Autodesk Fusion 360 part; units mm, degrees
(part 8 of 40)
  line L3316 (187.8528, 216.8887) -> (187.8788, 217.0208) construction
  line L3317 (187.8788, 217.0208) -> (187.8986, 217.1199) construction
  line L3318 (187.8986, 217.1199) -> (187.912, 217.186) construction
  line L3319 (187.912, 217.186) -> (187.9188, 217.2191) construction
  arc A105 (192.2105, 218.6136) -> (187.9188, 217.2191) centre (212.132, 150) ccw
  arc A106 (192.2105, 218.6136) -> (187.9188, 217.2191) centre (212.132, 150) ccw
  line L3320 (271.2762, 155.5428) -> (272.9005, 155.6951)
  spline S44 degree 5 poles (206.4369, 89.2315) (206.4341, 89.2007) (206.4291, 89.1391) (206.4242, 89.0467) (206.4223, 88.9234) (206.4264, 88.769) (206.4351, 88.6144) (206.4466, 88.4597) (206.4597, 88.305) (206.4737, 88.1502) (206.4889, 87.9955) (206.5055, 87.8407) (206.524, 87.686) (206.5449, 87.5312) (206.5679, 87.3765) (206.593, 87.2218) (206.6199, 87.0671) (206.6482, 86.9125) (206.6778, 86.7579) (206.7087, 86.6034) (206.7407, 86.4489) (206.7741, 86.2945) (206.8088, 86.1402) (206.8449, 85.986) (206.8823, 85.8318) (206.9211, 85.6778) (206.9611, 85.5238) (207.0023, 85.3699) (207.0447, 85.2161) (207.0881, 85.0624) (207.1327, 84.9088) (207.1784, 84.7553) (207.2252, 84.602) (207.2731, 84.4487) (207.3221, 84.2956) (207.3721, 84.1426) (207.4233, 83.9897) (207.4754, 83.8369) (207.5285, 83.6842) (207.5827, 83.5317) (207.6378, 83.3794) (207.694, 83.2271) (207.751, 83.075) (207.8091, 82.923) (207.8681, 82.7712) (207.9281, 82.6196) (207.989, 82.468) (208.0508, 82.3167) (208.1135, 82.1655) (208.1772, 82.0144) (208.2417, 81.8635) (208.3071, 81.7128) (208.3735, 81.5622) (208.4407, 81.4118) (208.5087, 81.2616) (208.5777, 81.1115) (208.6474, 80.9616) (208.7181, 80.8119) (208.7895, 80.6624) (208.8619, 80.513) (208.935, 80.3638) (209.009, 80.2148) (209.0838, 80.066) (209.1594, 79.9174) (209.2358, 79.7689) (209.313, 79.6207) (209.391, 79.4726) (209.4698, 79.3248) (209.5494, 79.1771) (209.6297, 79.0297) (209.7109, 78.8824) (209.7764, 78.7648) (209.8259, 78.6766) (209.8591, 78.6179) (209.8757, 78.5885) knots 0 0 0 0 0 0 0.01428571 0.02857143 0.04285714 0.05714286 0.07142857 0.08571429 0.1 0.11428571 0.12857143 0.14285714 0.15714286 0.17142857 0.18571429 0.2 0.21428571 0.22857143 0.24285714 0.25714286 0.27142857 0.28571429 0.3 0.31428571 0.32857143 0.34285714 0.35714286 0.37142857 0.38571429 0.4 0.41428571 0.42857143 0.44285714 0.45714286 0.47142857 0.48571429 0.5 0.51428571 0.52857143 0.54285714 0.55714286 0.57142857 0.58571429 0.6 0.61428571 0.62857143 0.64285714 0.65714286 0.67142857 0.68571429 0.7 0.71428571 0.72857143 0.74285714 0.75714286 0.77142857 0.78571429 0.8 0.81428571 0.82857143 0.84285714 0.85714286 0.87142857 0.88571429 0.9 0.91428571 0.92857143 0.94285714 0.95714286 0.97142857 0.98571429 1 1 1 1 1 1
  line L3321 (206.4369, 89.2315) -> (206.4341, 89.2007) construction
  line L3322 (206.4341, 89.2007) -> (206.4291, 89.1391) construction
  line L3323 (206.4291, 89.1391) -> (206.4242, 89.0467) construction
  line L3324 (206.4242, 89.0467) -> (206.4223, 88.9234) construction
  line L3325 (206.4223, 88.9234) -> (206.4264, 88.769) construction
  line L3326 (206.4264, 88.769) -> (206.4351, 88.6144) construction
  line L3327 (206.4351, 88.6144) -> (206.4466, 88.4597) construction
  line L3328 (206.4466, 88.4597) -> (206.4597, 88.305) construction
  line L3329 (206.4597, 88.305) -> (206.4737, 88.1502) construction
  line L3330 (206.4737, 88.1502) -> (206.4889, 87.9955) construction
  line L3331 (206.4889, 87.9955) -> (206.5055, 87.8407) construction
  line L3332 (206.5055, 87.8407) -> (206.524, 87.686) construction
  line L3333 (206.524, 87.686) -> (206.5449, 87.5312) construction
  line L3334 (206.5449, 87.5312) -> (206.5679, 87.3765) construction
  line L3335 (206.5679, 87.3765) -> (206.593, 87.2218) construction
  line L3336 (206.593, 87.2218) -> (206.6199, 87.0671) construction
  line L3337 (206.6199, 87.0671) -> (206.6482, 86.9125) construction
  line L3338 (206.6482, 86.9125) -> (206.6778, 86.7579) construction
  line L3339 (206.6778, 86.7579) -> (206.7087, 86.6034) construction
  line L3340 (206.7087, 86.6034) -> (206.7407, 86.4489) construction
  line L3341 (206.7407, 86.4489) -> (206.7741, 86.2945) construction
  line L3342 (206.7741, 86.2945) -> (206.8088, 86.1402) construction
  line L3343 (206.8088, 86.1402) -> (206.8449, 85.986) construction
  line L3344 (206.8449, 85.986) -> (206.8823, 85.8318) construction
  line L3345 (206.8823, 85.8318) -> (206.9211, 85.6778) construction
  line L3346 (206.9211, 85.6778) -> (206.9611, 85.5238) construction
  line L3347 (206.9611, 85.5238) -> (207.0023, 85.3699) construction
  line L3348 (207.0023, 85.3699) -> (207.0447, 85.2161) construction
  line L3349 (207.0447, 85.2161) -> (207.0881, 85.0624) construction
  line L3350 (207.0881, 85.0624) -> (207.1327, 84.9088) construction
  line L3351 (207.1327, 84.9088) -> (207.1784, 84.7553) construction
  line L3352 (207.1784, 84.7553) -> (207.2252, 84.602) construction
  line L3353 (207.2252, 84.602) -> (207.2731, 84.4487) construction
  line L3354 (207.2731, 84.4487) -> (207.3221, 84.2956) construction
  line L3355 (207.3221, 84.2956) -> (207.3721, 84.1426) construction
  line L3356 (207.3721, 84.1426) -> (207.4233, 83.9897) construction
  line L3357 (207.4233, 83.9897) -> (207.4754, 83.8369) construction
  line L3358 (207.4754, 83.8369) -> (207.5285, 83.6842) construction
  line L3359 (207.5285, 83.6842) -> (207.5827, 83.5317) construction
  line L3360 (207.5827, 83.5317) -> (207.6378, 83.3794) construction
  line L3361 (207.6378, 83.3794) -> (207.694, 83.2271) construction
  line L3362 (207.694, 83.2271) -> (207.751, 83.075) construction
  line L3363 (207.751, 83.075) -> (207.8091, 82.923) construction
  line L3364 (207.8091, 82.923) -> (207.8681, 82.7712) construction
  line L3365 (207.8681, 82.7712) -> (207.9281, 82.6196) construction
  line L3366 (207.9281, 82.6196) -> (207.989, 82.468) construction
  line L3367 (207.989, 82.468) -> (208.0508, 82.3167) construction
  line L3368 (208.0508, 82.3167) -> (208.1135, 82.1655) construction
  line L3369 (208.1135, 82.1655) -> (208.1772, 82.0144) construction
  line L3370 (208.1772, 82.0144) -> (208.2417, 81.8635) construction
  line L3371 (208.2417, 81.8635) -> (208.3071, 81.7128) construction
  line L3372 (208.3071, 81.7128) -> (208.3735, 81.5622) construction
  line L3373 (208.3735, 81.5622) -> (208.4407, 81.4118) construction
  line L3374 (208.4407, 81.4118) -> (208.5087, 81.2616) construction
  line L3375 (208.5087, 81.2616) -> (208.5777, 81.1115) construction
  line L3376 (208.5777, 81.1115) -> (208.6474, 80.9616) construction
  line L3377 (208.6474, 80.9616) -> (208.7181, 80.8119) construction
  line L3378 (208.7181, 80.8119) -> (208.7895, 80.6624) construction
  line L3379 (208.7895, 80.6624) -> (208.8619, 80.513) construction
  line L3380 (208.8619, 80.513) -> (208.935, 80.3638) construction
  line L3381 (208.935, 80.3638) -> (209.009, 80.2148) construction
  line L3382 (209.009, 80.2148) -> (209.0838, 80.066) construction
  line L3383 (209.0838, 80.066) -> (209.1594, 79.9174) construction
  line L3384 (209.1594, 79.9174) -> (209.2358, 79.7689) construction
  line L3385 (209.2358, 79.7689) -> (209.313, 79.6207) construction
  line L3386 (209.313, 79.6207) -> (209.391, 79.4726) construction
  line L3387 (209.391, 79.4726) -> (209.4698, 79.3248) construction
  line L3388 (209.4698, 79.3248) -> (209.5494, 79.1771) construction
  line L3389 (209.5494, 79.1771) -> (209.6297, 79.0297) construction
  line L3390 (209.6297, 79.0297) -> (209.7109, 78.8824) construction
  line L3391 (209.7109, 78.8824) -> (209.7764, 78.7648) construction
  line L3392 (209.7764, 78.7648) -> (209.8259, 78.6766) construction
  line L3393 (209.8259, 78.6766) -> (209.8591, 78.6179) construction
  line L3394 (209.8591, 78.6179) -> (209.8757, 78.5885) construction
  spline S45 degree 5 poles (206.4369, 89.2315) (206.4341, 89.2007) (206.4291, 89.1391) (206.4242, 89.0467) (206.4223, 88.9234) (206.4264, 88.769) (206.4351, 88.6144) (206.4466, 88.4597) (206.4597, 88.305) (206.4737, 88.1502) (206.4889, 87.9955) (206.5055, 87.8407) (206.524, 87.686) (206.5449, 87.5312) (206.5679, 87.3765) (206.593, 87.2218) (206.6199, 87.0671) (206.6482, 86.9125) (206.6778, 86.7579) (206.7087, 86.6034) (206.7407, 86.4489) (206.7741, 86.2945) (206.8088, 86.1402) (206.8449, 85.986) (206.8823, 85.8318) (206.9211, 85.6778) (206.9611, 85.5238) (207.0023, 85.3699) (207.0447, 85.2161) (207.0881, 85.0624) (207.1327, 84.9088) (207.1784, 84.7553) (207.2252, 84.602) (207.2731, 84.4487) (207.3221, 84.2956) (207.3721, 84.1426) (207.4233, 83.9897) (207.4754, 83.8369) (207.5285, 83.6842) (207.5827, 83.5317) (207.6378, 83.3794) (207.694, 83.2271) (207.751, 83.075) (207.8091, 82.923) (207.8681, 82.7712) (207.9281, 82.6196) (207.989, 82.468) (208.0508, 82.3167) (208.1135, 82.1655) (208.1772, 82.0144) (208.2417, 81.8635) (208.3071, 81.7128) (208.3735, 81.5622) (208.4407, 81.4118) (208.5087, 81.2616) (208.5777, 81.1115) (208.6474, 80.9616) (208.7181, 80.8119) (208.7895, 80.6624) (208.8619, 80.513) (208.935, 80.3638) (209.009, 80.2148) (209.0838, 80.066) (209.1594, 79.9174) (209.2358, 79.7689) (209.313, 79.6207) (209.391, 79.4726) (209.4698, 79.3248) (209.5494, 79.1771) (209.6297, 79.0297) (209.7109, 78.8824) (209.7764, 78.7648) (209.8259, 78.6766) (209.8591, 78.6179) (209.8757, 78.5885) knots 0 0 0 0 0 0 0.01428571 0.02857143 0.04285714 0.05714286 0.07142857 0.08571429 0.1 0.11428571 0.12857143 0.14285714 0.15714286 0.17142857 0.18571429 0.2 0.21428571 0.22857143 0.24285714 0.25714286 0.27142857 0.28571429 0.3 0.31428571 0.32857143 0.34285714 0.35714286 0.37142857 0.38571429 0.4 0.41428571 0.42857143 0.44285714 0.45714286 0.47142857 0.48571429 0.5 0.51428571 0.52857143 0.54285714 0.55714286 0.57142857 0.58571429 0.6 0.61428571 0.62857143 0.64285714 0.65714286 0.67142857 0.68571429 0.7 0.71428571 0.72857143 0.74285714 0.75714286 0.77142857 0.78571429 0.8 0.81428571 0.82857143 0.84285714 0.85714286 0.87142857 0.88571429 0.9 0.91428571 0.92857143 0.94285714 0.95714286 0.97142857 0.98571429 1 1 1 1 1 1
  line L3395 (206.4369, 89.2315) -> (206.4341, 89.2007) construction
  line L3396 (206.4341, 89.2007) -> (206.4291, 89.1391) construction
  line L3397 (206.4291, 89.1391) -> (206.4242, 89.0467) construction
  line L3398 (206.4242, 89.0467) -> (206.4223, 88.9234) construction
  line L3399 (206.4223, 88.9234) -> (206.4264, 88.769) construction
  line L3400 (206.4264, 88.769) -> (206.4351, 88.6144) construction
  line L3401 (206.4351, 88.6144) -> (206.4466, 88.4597) construction
  line L3402 (206.4466, 88.4597) -> (206.4597, 88.305) construction
  line L3403 (206.4597, 88.305) -> (206.4737, 88.1502) construction
  line L3404 (206.4737, 88.1502) -> (206.4889, 87.9955) construction
  line L3405 (206.4889, 87.9955) -> (206.5055, 87.8407) construction
  line L3406 (206.5055, 87.8407) -> (206.524, 87.686) construction
  line L3407 (206.524, 87.686) -> (206.5449, 87.5312) construction
  line L3408 (206.5449, 87.5312) -> (206.5679, 87.3765) construction
  line L3409 (206.5679, 87.3765) -> (206.593, 87.2218) construction
  line L3410 (206.593, 87.2218) -> (206.6199, 87.0671) construction
  line L3411 (206.6199, 87.0671) -> (206.6482, 86.9125) construction
  line L3412 (206.6482, 86.9125) -> (206.6778, 86.7579) construction
  line L3413 (206.6778, 86.7579) -> (206.7087, 86.6034) construction
  line L3414 (206.7087, 86.6034) -> (206.7407, 86.4489) construction
  line L3415 (206.7407, 86.4489) -> (206.7741, 86.2945) construction
  line L3416 (206.7741, 86.2945) -> (206.8088, 86.1402) construction
  line L3417 (206.8088, 86.1402) -> (206.8449, 85.986) construction
  line L3418 (206.8449, 85.986) -> (206.8823, 85.8318) construction
  line L3419 (206.8823, 85.8318) -> (206.9211, 85.6778) construction
  line L3420 (206.9211, 85.6778) -> (206.9611, 85.5238) construction
  line L3421 (206.9611, 85.5238) -> (207.0023, 85.3699) construction
  line L3422 (207.0023, 85.3699) -> (207.0447, 85.2161) construction
  line L3423 (207.0447, 85.2161) -> (207.0881, 85.0624) construction
  line L3424 (207.0881, 85.0624) -> (207.1327, 84.9088) construction
  line L3425 (207.1327, 84.9088) -> (207.1784, 84.7553) construction
  line L3426 (207.1784, 84.7553) -> (207.2252, 84.602) construction
  line L3427 (207.2252, 84.602) -> (207.2731, 84.4487) construction
  line L3428 (207.2731, 84.4487) -> (207.3221, 84.2956) construction
  line L3429 (207.3221, 84.2956) -> (207.3721, 84.1426) construction
  line L3430 (207.3721, 84.1426) -> (207.4233, 83.9897) construction
  line L3431 (207.4233, 83.9897) -> (207.4754, 83.8369) construction
  line L3432 (207.4754, 83.8369) -> (207.5285, 83.6842) construction
  line L3433 (207.5285, 83.6842) -> (207.5827, 83.5317) construction
  line L3434 (207.5827, 83.5317) -> (207.6378, 83.3794) construction
  line L3435 (207.6378, 83.3794) -> (207.694, 83.2271) construction
  line L3436 (207.694, 83.2271) -> (207.751, 83.075) construction
  line L3437 (207.751, 83.075) -> (207.8091, 82.923) construction
  line L3438 (207.8091, 82.923) -> (207.8681, 82.7712) construction
  line L3439 (207.8681, 82.7712) -> (207.9281, 82.6196) construction
  line L3440 (207.9281, 82.6196) -> (207.989, 82.468) construction
  line L3441 (207.989, 82.468) -> (208.0508, 82.3167) construction
  line L3442 (208.0508, 82.3167) -> (208.1135, 82.1655) construction
  line L3443 (208.1135, 82.1655) -> (208.1772, 82.0144) construction
  line L3444 (208.1772, 82.0144) -> (208.2417, 81.8635) construction
  line L3445 (208.2417, 81.8635) -> (208.3071, 81.7128) construction
  line L3446 (208.3071, 81.7128) -> (208.3735, 81.5622) construction
  line L3447 (208.3735, 81.5622) -> (208.4407, 81.4118) construction
  line L3448 (208.4407, 81.4118) -> (208.5087, 81.2616) construction
  line L3449 (208.5087, 81.2616) -> (208.5777, 81.1115) construction
  line L3450 (208.5777, 81.1115) -> (208.6474, 80.9616) construction
  line L3451 (208.6474, 80.9616) -> (208.7181, 80.8119) construction
  line L3452 (208.7181, 80.8119) -> (208.7895, 80.6624) construction
  line L3453 (208.7895, 80.6624) -> (208.8619, 80.513) construction
  line L3454 (208.8619, 80.513) -> (208.935, 80.3638) construction
  line L3455 (208.935, 80.3638) -> (209.009, 80.2148) construction
  line L3456 (209.009, 80.2148) -> (209.0838, 80.066) construction
  line L3457 (209.0838, 80.066) -> (209.1594, 79.9174) construction
  line L3458 (209.1594, 79.9174) -> (209.2358, 79.7689) construction
  line L3459 (209.2358, 79.7689) -> (209.313, 79.6207) construction
  line L3460 (209.313, 79.6207) -> (209.391, 79.4726) construction
  line L3461 (209.391, 79.4726) -> (209.4698, 79.3248) construction
  line L3462 (209.4698, 79.3248) -> (209.5494, 79.1771) construction
  line L3463 (209.5494, 79.1771) -> (209.6297, 79.0297) construction
  line L3464 (209.6297, 79.0297) -> (209.7109, 78.8824) construction
  line L3465 (209.7109, 78.8824) -> (209.7764, 78.7648) construction
  line L3466 (209.7764, 78.7648) -> (209.8259, 78.6766) construction
  line L3467 (209.8259, 78.6766) -> (209.8591, 78.6179) construction
  line L3468 (209.8591, 78.6179) -> (209.8757, 78.5885) construction
  arc A107 (209.8757, 78.5885) -> (214.3883, 78.5885) centre (212.132, 150) ccw
  arc A108 (209.8757, 78.5885) -> (214.3883, 78.5885) centre (212.132, 150) ccw
  spline S46 degree 5 poles (252.4583, 104.1847) (252.4787, 104.1615) (252.5188, 104.1146) (252.5771, 104.0427) (252.6512, 103.944) (252.7386, 103.8167) (252.8224, 103.6865) (252.904, 103.5546) (252.9844, 103.4218) (253.064, 103.2883) (253.1427, 103.1542) (253.2203, 103.0193) (253.2962, 102.8832) (253.3703, 102.7457) (253.4426, 102.607) (253.5133, 102.4671) (253.5824, 102.3262) (253.6504, 102.1844) (253.7173, 102.0419) (253.7832, 101.8988) (253.848, 101.755) (253.9118, 101.6105) (253.9744, 101.4653) (254.0359, 101.3193) (254.0962, 101.1726) (254.1554, 101.0251) (254.2135, 100.877) (254.2706, 100.7283) (254.3267, 100.579) (254.3819, 100.4291) (254.4361, 100.2786) (254.4894, 100.1276) (254.5417, 99.976) (254.593, 99.8239) (254.6434, 99.6712) (254.6928, 99.518) (254.7414, 99.3642) (254.789, 99.21) (254.8357, 99.0553) (254.8815, 98.9001) (254.9265, 98.7444) (254.9706, 98.5882) (255.0138, 98.4316) (255.0561, 98.2745) (255.0976, 98.117) (255.1383, 97.9591) (255.1781, 97.8007) (255.217, 97.6419) (255.2551, 97.4827) (255.2924, 97.3231) (255.3289, 97.1631) (255.3646, 97.0027) (255.3994, 96.8419) (255.4335, 96.6807) (255.4667, 96.5191) (255.4992, 96.3572) (255.5308, 96.1949) (255.5617, 96.0323) (255.5917, 95.8693) (255.621, 95.706) (255.6495, 95.5423) (255.6773, 95.3783) (255.7043, 95.2139) (255.7304, 95.0492) (255.7559, 94.8842) (255.7806, 94.7189) (255.8045, 94.5533) (255.8276, 94.3874) (255.85, 94.2211) (255.8717, 94.0546) (255.8926, 93.8878) (255.9087, 93.7541) (255.9205, 93.6537) (255.9282, 93.5867) (255.932, 93.5531) knots 0 0 0 0 0 0 0.01428571 0.02857143 0.04285714 0.05714286 0.07142857 0.08571429 0.1 0.11428571 0.12857143 0.14285714 0.15714286 0.17142857 0.18571429 0.2 0.21428571 0.22857143 0.24285714 0.25714286 0.27142857 0.28571429 0.3 0.31428571 0.32857143 0.34285714 0.35714286 0.37142857 0.38571429 0.4 0.41428571 0.42857143 0.44285714 0.45714286 0.47142857 0.48571429 0.5 0.51428571 0.52857143 0.54285714 0.55714286 0.57142857 0.58571429 0.6 0.61428571 0.62857143 0.64285714 0.65714286 0.67142857 0.68571429 0.7 0.71428571 0.72857143 0.74285714 0.75714286 0.77142857 0.78571429 0.8 0.81428571 0.82857143 0.84285714 0.85714286 0.87142857 0.88571429 0.9 0.91428571 0.92857143 0.94285714 0.95714286 0.97142857 0.98571429 1 1 1 1 1 1
  line L3469 (252.4583, 104.1847) -> (252.4787, 104.1615) construction
  line L3470 (252.4787, 104.1615) -> (252.5188, 104.1146) construction
  line L3471 (252.5188, 104.1146) -> (252.5771, 104.0427) construction
  line L3472 (252.5771, 104.0427) -> (252.6512, 103.944) construction
  line L3473 (252.6512, 103.944) -> (252.7386, 103.8167) construction
  line L3474 (252.7386, 103.8167) -> (252.8224, 103.6865) construction
  line L3475 (252.8224, 103.6865) -> (252.904, 103.5546) construction
  line L3476 (252.904, 103.5546) -> (252.9844, 103.4218) construction
  line L3477 (252.9844, 103.4218) -> (253.064, 103.2883) construction
  line L3478 (253.064, 103.2883) -> (253.1427, 103.1542) construction
  line L3479 (253.1427, 103.1542) -> (253.2203, 103.0193) construction
  line L3480 (253.2203, 103.0193) -> (253.2962, 102.8832) construction
  line L3481 (253.2962, 102.8832) -> (253.3703, 102.7457) construction
  line L3482 (253.3703, 102.7457) -> (253.4426, 102.607) construction
  line L3483 (253.4426, 102.607) -> (253.5133, 102.4671) construction
  line L3484 (253.5133, 102.4671) -> (253.5824, 102.3262) construction
  line L3485 (253.5824, 102.3262) -> (253.6504, 102.1844) construction
  line L3486 (253.6504, 102.1844) -> (253.7173, 102.0419) construction
  line L3487 (253.7173, 102.0419) -> (253.7832, 101.8988) construction
  line L3488 (253.7832, 101.8988) -> (253.848, 101.755) construction
  line L3489 (253.848, 101.755) -> (253.9118, 101.6105) construction
  line L3490 (253.9118, 101.6105) -> (253.9744, 101.4653) construction
  line L3491 (253.9744, 101.4653) -> (254.0359, 101.3193) construction
  line L3492 (254.0359, 101.3193) -> (254.0962, 101.1726) construction
  line L3493 (254.0962, 101.1726) -> (254.1554, 101.0251) construction
  line L3494 (254.1554, 101.0251) -> (254.2135, 100.877) construction
  line L3495 (254.2135, 100.877) -> (254.2706, 100.7283) construction
  line L3496 (254.2706, 100.7283) -> (254.3267, 100.579) construction
  line L3497 (254.3267, 100.579) -> (254.3819, 100.4291) construction
  line L3498 (254.3819, 100.4291) -> (254.4361, 100.2786) construction
  line L3499 (254.4361, 100.2786) -> (254.4894, 100.1276) construction
  line L3500 (254.4894, 100.1276) -> (254.5417, 99.976) construction
  line L3501 (254.5417, 99.976) -> (254.593, 99.8239) construction
  line L3502 (254.593, 99.8239) -> (254.6434, 99.6712) construction
  line L3503 (254.6434, 99.6712) -> (254.6928, 99.518) construction
  line L3504 (254.6928, 99.518) -> (254.7414, 99.3642) construction
  line L3505 (254.7414, 99.3642) -> (254.789, 99.21) construction
  line L3506 (254.789, 99.21) -> (254.8357, 99.0553) construction
  line L3507 (254.8357, 99.0553) -> (254.8815, 98.9001) construction
  line L3508 (254.8815, 98.9001) -> (254.9265, 98.7444) construction
  line L3509 (254.9265, 98.7444) -> (254.9706, 98.5882) construction
  line L3510 (254.9706, 98.5882) -> (255.0138, 98.4316) construction
  line L3511 (255.0138, 98.4316) -> (255.0561, 98.2745) construction
  line L3512 (255.0561, 98.2745) -> (255.0976, 98.117) construction
  line L3513 (255.0976, 98.117) -> (255.1383, 97.9591) construction
  line L3514 (255.1383, 97.9591) -> (255.1781, 97.8007) construction
  line L3515 (255.1781, 97.8007) -> (255.217, 97.6419) construction
  line L3516 (255.217, 97.6419) -> (255.2551, 97.4827) construction
  line L3517 (255.2551, 97.4827) -> (255.2924, 97.3231) construction
  line L3518 (255.2924, 97.3231) -> (255.3289, 97.1631) construction
  line L3519 (255.3289, 97.1631) -> (255.3646, 97.0027) construction
  line L3520 (255.3646, 97.0027) -> (255.3994, 96.8419) construction
  line L3521 (255.3994, 96.8419) -> (255.4335, 96.6807) construction
  line L3522 (255.4335, 96.6807) -> (255.4667, 96.5191) construction
  line L3523 (255.4667, 96.5191) -> (255.4992, 96.3572) construction
  line L3524 (255.4992, 96.3572) -> (255.5308, 96.1949) construction
  line L3525 (255.5308, 96.1949) -> (255.5617, 96.0323) construction
  line L3526 (255.5617, 96.0323) -> (255.5917, 95.8693) construction
  line L3527 (255.5917, 95.8693) -> (255.621, 95.706) construction
  line L3528 (255.621, 95.706) -> (255.6495, 95.5423) construction
  line L3529 (255.6495, 95.5423) -> (255.6773, 95.3783) construction
  line L3530 (255.6773, 95.3783) -> (255.7043, 95.2139) construction
  line L3531 (255.7043, 95.2139) -> (255.7304, 95.0492) construction
  line L3532 (255.7304, 95.0492) -> (255.7559, 94.8842) construction
  line L3533 (255.7559, 94.8842) -> (255.7806, 94.7189) construction
  line L3534 (255.7806, 94.7189) -> (255.8045, 94.5533) construction
  line L3535 (255.8045, 94.5533) -> (255.8276, 94.3874) construction
  line L3536 (255.8276, 94.3874) -> (255.85, 94.2211) construction
  line L3537 (255.85, 94.2211) -> (255.8717, 94.0546) construction
  line L3538 (255.8717, 94.0546) -> (255.8926, 93.8878) construction
  line L3539 (255.8926, 93.8878) -> (255.9087, 93.7541) construction
  line L3540 (255.9087, 93.7541) -> (255.9205, 93.6537) construction
  line L3541 (255.9205, 93.6537) -> (255.9282, 93.5867) construction
  line L3542 (255.9282, 93.5867) -> (255.932, 93.5531) construction
  spline S47 degree 5 poles (271.6862, 163.3622) (271.7163, 163.369) (271.7764, 163.3833) (271.8658, 163.4071) (271.9837, 163.4435) (272.1293, 163.4951) (272.2736, 163.5511) (272.4172, 163.6099) (272.5603, 163.6701) (272.7031, 163.7313) (272.8456, 163.7935) (272.9877, 163.8571) (273.1291, 163.9226) (273.2699, 163.9902) (273.4099, 164.06) (273.5493, 164.1316) (273.6881, 164.205) (273.8264, 164.2797) (273.9642, 164.3557) (274.1017, 164.4327) (274.2387, 164.5109) (274.3752, 164.5904) (274.5112, 164.6711) (274.6468, 164.753) (274.7818, 164.8363) (274.9163, 164.9208) (275.0504, 165.0064) (275.184, 165.0932) (275.3172, 165.181) (275.45, 165.2698) (275.5823, 165.3597) (275.7141, 165.4506) (275.8455, 165.5425) (275.9765, 165.6354) (276.107, 165.7293) (276.237, 165.8242) (276.3666, 165.92) (276.4958, 166.0168) (276.6246, 166.1146) (276.7529, 166.2132) (276.8808, 166.3127) (277.0082, 166.4131) (277.1352, 166.5144) (277.2618, 166.6166) (277.388, 166.7196) (277.5137, 166.8235) (277.639, 166.9283) (277.7638, 167.0338) (277.8882, 167.1402) (278.0122, 167.2474) (278.1358, 167.3555) (278.2589, 167.4643) (278.3817, 167.5739) (278.5039, 167.6842) (278.6258, 167.7954) (278.7472, 167.9073) (278.8682, 168.02) (278.9888, 168.1335) (279.1089, 168.2477) (279.2286, 168.3626) (279.3479, 168.4782) (279.4667, 168.5946) (279.5851, 168.7118) (279.7031, 168.8296) (279.8207, 168.9481) (279.9378, 169.0674) (280.0545, 169.1873) (280.1708, 169.3079) (280.2866, 169.4293) (280.402, 169.5512) (280.517, 169.6739) (280.6087, 169.7726) (280.6772, 169.8469) (280.7228, 169.8966) (280.7456, 169.9215) knots 0 0 0 0 0 0 0.01428571 0.02857143 0.04285714 0.05714286 0.07142857 0.08571429 0.1 0.11428571 0.12857143 0.14285714 0.15714286 0.17142857 0.18571429 0.2 0.21428571 0.22857143 0.24285714 0.25714286 0.27142857 0.28571429 0.3 0.31428571 0.32857143 0.34285714 0.35714286 0.37142857 0.38571429 0.4 0.41428571 0.42857143 0.44285714 0.45714286 0.47142857 0.48571429 0.5 0.51428571 0.52857143 0.54285714 0.55714286 0.57142857 0.58571429 0.6 0.61428571 0.62857143 0.64285714 0.65714286 0.67142857 0.68571429 0.7 0.71428571 0.72857143 0.74285714 0.75714286 0.77142857 0.78571429 0.8 0.81428571 0.82857143 0.84285714 0.85714286 0.87142857 0.88571429 0.9 0.91428571 0.92857143 0.94285714 0.95714286 0.97142857 0.98571429 1 1 1 1 1 1
  line L3543 (271.6862, 163.3622) -> (271.7163, 163.369) construction
  line L3544 (271.7163, 163.369) -> (271.7764, 163.3833) construction
  line L3545 (271.7764, 163.3833) -> (271.8658, 163.4071) construction
  line L3546 (271.8658, 163.4071) -> (271.9837, 163.4435) construction
  line L3547 (271.9837, 163.4435) -> (272.1293, 163.4951) construction
  line L3548 (272.1293, 163.4951) -> (272.2736, 163.5511) construction
  line L3549 (272.2736, 163.5511) -> (272.4172, 163.6099) construction
  line L3550 (272.4172, 163.6099) -> (272.5603, 163.6701) construction
  line L3551 (272.5603, 163.6701) -> (272.7031, 163.7313) construction
  line L3552 (272.7031, 163.7313) -> (272.8456, 163.7935) construction
  line L3553 (272.8456, 163.7935) -> (272.9877, 163.8571) construction
  line L3554 (272.9877, 163.8571) -> (273.1291, 163.9226) construction
  line L3555 (273.1291, 163.9226) -> (273.2699, 163.9902) construction
  line L3556 (273.2699, 163.9902) -> (273.4099, 164.06) construction
  line L3557 (273.4099, 164.06) -> (273.5493, 164.1316) construction
  line L3558 (273.5493, 164.1316) -> (273.6881, 164.205) construction
  line L3559 (273.6881, 164.205) -> (273.8264, 164.2797) construction
  line L3560 (273.8264, 164.2797) -> (273.9642, 164.3557) construction
  line L3561 (273.9642, 164.3557) -> (274.1017, 164.4327) construction
  line L3562 (274.1017, 164.4327) -> (274.2387, 164.5109) construction
  line L3563 (274.2387, 164.5109) -> (274.3752, 164.5904) construction
  line L3564 (274.3752, 164.5904) -> (274.5112, 164.6711) construction
  line L3565 (274.5112, 164.6711) -> (274.6468, 164.753) construction
  line L3566 (274.6468, 164.753) -> (274.7818, 164.8363) construction
  line L3567 (274.7818, 164.8363) -> (274.9163, 164.9208) construction
  line L3568 (274.9163, 164.9208) -> (275.0504, 165.0064) construction
  line L3569 (275.0504, 165.0064) -> (275.184, 165.0932) construction
  line L3570 (275.184, 165.0932) -> (275.3172, 165.181) construction
  line L3571 (275.3172, 165.181) -> (275.45, 165.2698) construction
  line L3572 (275.45, 165.2698) -> (275.5823, 165.3597) construction
  line L3573 (275.5823, 165.3597) -> (275.7141, 165.4506) construction
  line L3574 (275.7141, 165.4506) -> (275.8455, 165.5425) construction
  line L3575 (275.8455, 165.5425) -> (275.9765, 165.6354) construction
  line L3576 (275.9765, 165.6354) -> (276.107, 165.7293) construction
  line L3577 (276.107, 165.7293) -> (276.237, 165.8242) construction
  line L3578 (276.237, 165.8242) -> (276.3666, 165.92) construction
  line L3579 (276.3666, 165.92) -> (276.4958, 166.0168) construction
  line L3580 (276.4958, 166.0168) -> (276.6246, 166.1146) construction
  line L3581 (276.6246, 166.1146) -> (276.7529, 166.2132) construction
  line L3582 (276.7529, 166.2132) -> (276.8808, 166.3127) construction
  line L3583 (276.8808, 166.3127) -> (277.0082, 166.4131) construction
  line L3584 (277.0082, 166.4131) -> (277.1352, 166.5144) construction
  line L3585 (277.1352, 166.5144) -> (277.2618, 166.6166) construction
  line L3586 (277.2618, 166.6166) -> (277.388, 166.7196) construction
  line L3587 (277.388, 166.7196) -> (277.5137, 166.8235) construction
  line L3588 (277.5137, 166.8235) -> (277.639, 166.9283) construction
  line L3589 (277.639, 166.9283) -> (277.7638, 167.0338) construction
  line L3590 (277.7638, 167.0338) -> (277.8882, 167.1402) construction
  line L3591 (277.8882, 167.1402) -> (278.0122, 167.2474) construction
  line L3592 (278.0122, 167.2474) -> (278.1358, 167.3555) construction
  line L3593 (278.1358, 167.3555) -> (278.2589, 167.4643) construction
  line L3594 (278.2589, 167.4643) -> (278.3817, 167.5739) construction
  line L3595 (278.3817, 167.5739) -> (278.5039, 167.6842) construction
  line L3596 (278.5039, 167.6842) -> (278.6258, 167.7954) construction
  line L3597 (278.6258, 167.7954) -> (278.7472, 167.9073) construction
  line L3598 (278.7472, 167.9073) -> (278.8682, 168.02) construction
  line L3599 (278.8682, 168.02) -> (278.9888, 168.1335) construction
  line L3600 (278.9888, 168.1335) -> (279.1089, 168.2477) construction
  line L3601 (279.1089, 168.2477) -> (279.2286, 168.3626) construction
  line L3602 (279.2286, 168.3626) -> (279.3479, 168.4782) construction
  line L3603 (279.3479, 168.4782) -> (279.4667, 168.5946) construction
  line L3604 (279.4667, 168.5946) -> (279.5851, 168.7118) construction
  line L3605 (279.5851, 168.7118) -> (279.7031, 168.8296) construction
  line L3606 (279.7031, 168.8296) -> (279.8207, 168.9481) construction
  line L3607 (279.8207, 168.9481) -> (279.9378, 169.0674) construction
  line L3608 (279.9378, 169.0674) -> (280.0545, 169.1873) construction
  line L3609 (280.0545, 169.1873) -> (280.1708, 169.3079) construction
  line L3610 (280.1708, 169.3079) -> (280.2866, 169.4293) construction
  line L3611 (280.2866, 169.4293) -> (280.402, 169.5512) construction
  line L3612 (280.402, 169.5512) -> (280.517, 169.6739) construction
  line L3613 (280.517, 169.6739) -> (280.6087, 169.7726) construction
  line L3614 (280.6087, 169.7726) -> (280.6772, 169.8469) construction
  line L3615 (280.6772, 169.8469) -> (280.7228, 169.8966) construction
  line L3616 (280.7228, 169.8966) -> (280.7456, 169.9215) construction
  arc A109 (269.1057, 157.2806) -> (271.2762, 155.5428) centre (271.0895, 157.5341) ccw
  spline S48 degree 5 poles (272.9005, 155.6951) (272.9313, 155.6979) (272.9929, 155.7029) (273.0853, 155.7078) (273.2086, 155.7097) (273.363, 155.7056) (273.5176, 155.6969) (273.6723, 155.6854) (273.827, 155.6723) (273.9818, 155.6583) (274.1365, 155.6431) (274.2913, 155.6265) (274.446, 155.608) (274.6008, 155.5871) (274.7555, 155.5641) (274.9102, 155.539) (275.0649, 155.5121) (275.2195, 155.4838) (275.3741, 155.4542) (275.5286, 155.4233) (275.6831, 155.3913) (275.8375, 155.3579) (275.9918, 155.3232) (276.146, 155.2871) (276.3002, 155.2497) (276.4542, 155.2109) (276.6082, 155.1709) (276.7621, 155.1297) (276.9159, 155.0873) (277.0696, 155.0439) (277.2232, 154.9993) (277.3767, 154.9536) (277.53, 154.9068) (277.6833, 154.8589) (277.8364, 154.8099) (277.9894, 154.7599) (278.1423, 154.7087) (278.2951, 154.6566) (278.4478, 154.6035) (278.6003, 154.5493) (278.7526, 154.4942) (278.9049, 154.438) (279.057, 154.381) (279.209, 154.3229) (279.3608, 154.2639) (279.5124, 154.2039) (279.664, 154.143) (279.8153, 154.0812) (279.9665, 154.0185) (280.1176, 153.9548) (280.2685, 153.8903) (280.4192, 153.8249) (280.5698, 153.7585) (280.7202, 153.6913) (280.8704, 153.6233) (281.0205, 153.5543) (281.1704, 153.4846) (281.3201, 153.4139) (281.4696, 153.3425) (281.619, 153.2701) (281.7682, 153.197) (281.9172, 153.123) (282.066, 153.0482) (282.2146, 152.9726) (282.3631, 152.8962) (282.5113, 152.819) (282.6594, 152.741) (282.8072, 152.6622) (282.9549, 152.5826) (283.1023, 152.5023) (283.2496, 152.4211) (283.3672, 152.3556) (283.4554, 152.3061) (283.5141, 152.2729) (283.5435, 152.2563) knots 0 0 0 0 0 0 0.01428571 0.02857143 0.04285714 0.05714286 0.07142857 0.08571429 0.1 0.11428571 0.12857143 0.14285714 0.15714286 0.17142857 0.18571429 0.2 0.21428571 0.22857143 0.24285714 0.25714286 0.27142857 0.28571429 0.3 0.31428571 0.32857143 0.34285714 0.35714286 0.37142857 0.38571429 0.4 0.41428571 0.42857143 0.44285714 0.45714286 0.47142857 0.48571429 0.5 0.51428571 0.52857143 0.54285714 0.55714286 0.57142857 0.58571429 0.6 0.61428571 0.62857143 0.64285714 0.65714286 0.67142857 0.68571429 0.7 0.71428571 0.72857143 0.74285714 0.75714286 0.77142857 0.78571429 0.8 0.81428571 0.82857143 0.84285714 0.85714286 0.87142857 0.88571429 0.9 0.91428571 0.92857143 0.94285714 0.95714286 0.97142857 0.98571429 1 1 1 1 1 1
  line L3617 (272.9005, 155.6951) -> (272.9313, 155.6979) construction
  line L3618 (272.9313, 155.6979) -> (272.9929, 155.7029) construction
  line L3619 (272.9929, 155.7029) -> (273.0853, 155.7078) construction
  line L3620 (273.0853, 155.7078) -> (273.2086, 155.7097) construction
  line L3621 (273.2086, 155.7097) -> (273.363, 155.7056) construction
  line L3622 (273.363, 155.7056) -> (273.5176, 155.6969) construction
  line L3623 (273.5176, 155.6969) -> (273.6723, 155.6854) construction
  line L3624 (273.6723, 155.6854) -> (273.827, 155.6723) construction
  line L3625 (273.827, 155.6723) -> (273.9818, 155.6583) construction
  line L3626 (273.9818, 155.6583) -> (274.1365, 155.6431) construction
  line L3627 (274.1365, 155.6431) -> (274.2913, 155.6265) construction
  line L3628 (274.2913, 155.6265) -> (274.446, 155.608) construction
  line L3629 (274.446, 155.608) -> (274.6008, 155.5871) construction
  line L3630 (274.6008, 155.5871) -> (274.7555, 155.5641) construction
  line L3631 (274.7555, 155.5641) -> (274.9102, 155.539) construction
  line L3632 (274.9102, 155.539) -> (275.0649, 155.5121) construction
  line L3633 (275.0649, 155.5121) -> (275.2195, 155.4838) construction
  line L3634 (275.2195, 155.4838) -> (275.3741, 155.4542) construction
  line L3635 (275.3741, 155.4542) -> (275.5286, 155.4233) construction
  line L3636 (275.5286, 155.4233) -> (275.6831, 155.3913) construction
  line L3637 (275.6831, 155.3913) -> (275.8375, 155.3579) construction
  line L3638 (275.8375, 155.3579) -> (275.9918, 155.3232) construction
  line L3639 (275.9918, 155.3232) -> (276.146, 155.2871) construction
  line L3640 (276.146, 155.2871) -> (276.3002, 155.2497) construction
  line L3641 (276.3002, 155.2497) -> (276.4542, 155.2109) construction
  line L3642 (276.4542, 155.2109) -> (276.6082, 155.1709) construction
  line L3643 (276.6082, 155.1709) -> (276.7621, 155.1297) construction
  line L3644 (276.7621, 155.1297) -> (276.9159, 155.0873) construction
  line L3645 (276.9159, 155.0873) -> (277.0696, 155.0439) construction
  line L3646 (277.0696, 155.0439) -> (277.2232, 154.9993) construction
  line L3647 (277.2232, 154.9993) -> (277.3767, 154.9536) construction
  line L3648 (277.3767, 154.9536) -> (277.53, 154.9068) construction
  line L3649 (277.53, 154.9068) -> (277.6833, 154.8589) construction
  line L3650 (277.6833, 154.8589) -> (277.8364, 154.8099) construction
  line L3651 (277.8364, 154.8099) -> (277.9894, 154.7599) construction
  line L3652 (277.9894, 154.7599) -> (278.1423, 154.7087) construction
  line L3653 (278.1423, 154.7087) -> (278.2951, 154.6566) construction
  line L3654 (278.2951, 154.6566) -> (278.4478, 154.6035) construction
  line L3655 (278.4478, 154.6035) -> (278.6003, 154.5493) construction
  line L3656 (278.6003, 154.5493) -> (278.7526, 154.4942) construction
  line L3657 (278.7526, 154.4942) -> (278.9049, 154.438) construction
  line L3658 (278.9049, 154.438) -> (279.057, 154.381) construction
  line L3659 (279.057, 154.381) -> (279.209, 154.3229) construction
  line L3660 (279.209, 154.3229) -> (279.3608, 154.2639) construction
  line L3661 (279.3608, 154.2639) -> (279.5124, 154.2039) construction
  line L3662 (279.5124, 154.2039) -> (279.664, 154.143) construction
  line L3663 (279.664, 154.143) -> (279.8153, 154.0812) construction
  line L3664 (279.8153, 154.0812) -> (279.9665, 154.0185) construction
  line L3665 (279.9665, 154.0185) -> (280.1176, 153.9548) construction
  line L3666 (280.1176, 153.9548) -> (280.2685, 153.8903) construction
  line L3667 (280.2685, 153.8903) -> (280.4192, 153.8249) construction
  line L3668 (280.4192, 153.8249) -> (280.5698, 153.7585) construction
  line L3669 (280.5698, 153.7585) -> (280.7202, 153.6913) construction
  line L3670 (280.7202, 153.6913) -> (280.8704, 153.6233) construction
  line L3671 (280.8704, 153.6233) -> (281.0205, 153.5543) construction
  line L3672 (281.0205, 153.5543) -> (281.1704, 153.4846) construction
  line L3673 (281.1704, 153.4846) -> (281.3201, 153.4139) construction
  line L3674 (281.3201, 153.4139) -> (281.4696, 153.3425) construction
  line L3675 (281.4696, 153.3425) -> (281.619, 153.2701) construction
  line L3676 (281.619, 153.2701) -> (281.7682, 153.197) construction
  line L3677 (281.7682, 153.197) -> (281.9172, 153.123) construction
  line L3678 (281.9172, 153.123) -> (282.066, 153.0482) construction
  line L3679 (282.066, 153.0482) -> (282.2146, 152.9726) construction
  line L3680 (282.2146, 152.9726) -> (282.3631, 152.8962) construction
  line L3681 (282.3631, 152.8962) -> (282.5113, 152.819) construction
  line L3682 (282.5113, 152.819) -> (282.6594, 152.741) construction
  line L3683 (282.6594, 152.741) -> (282.8072, 152.6622) construction
  line L3684 (282.8072, 152.6622) -> (282.9549, 152.5826) construction
  line L3685 (282.9549, 152.5826) -> (283.1023, 152.5023) construction
  line L3686 (283.1023, 152.5023) -> (283.2496, 152.4211) construction
  line L3687 (283.2496, 152.4211) -> (283.3672, 152.3556) construction
  line L3688 (283.3672, 152.3556) -> (283.4554, 152.3061) construction
  line L3689 (283.4554, 152.3061) -> (283.5141, 152.2729) construction
  line L3690 (283.5141, 152.2729) -> (283.5435, 152.2563) construction
  spline S49 degree 5 poles (271.6862, 163.3622) (271.7163, 163.369) (271.7764, 163.3833) (271.8658, 163.4071) (271.9837, 163.4435) (272.1293, 163.4951) (272.2736, 163.5511) (272.4172, 163.6099) (272.5603, 163.6701) (272.7031, 163.7313) (272.8456, 163.7935) (272.9877, 163.8571) (273.1291, 163.9226) (273.2699, 163.9902) (273.4099, 164.06) (273.5493, 164.1316) (273.6881, 164.205) (273.8264, 164.2797) (273.9642, 164.3557) (274.1017, 164.4327) (274.2387, 164.5109) (274.3752, 164.5904) (274.5112, 164.6711) (274.6468, 164.753) (274.7818, 164.8363) (274.9163, 164.9208) (275.0504, 165.0064) (275.184, 165.0932) (275.3172, 165.181) (275.45, 165.2698) (275.5823, 165.3597) (275.7141, 165.4506) (275.8455, 165.5425) (275.9765, 165.6354) (276.107, 165.7293) (276.237, 165.8242) (276.3666, 165.92) (276.4958, 166.0168) (276.6246, 166.1146) (276.7529, 166.2132) (276.8808, 166.3127) (277.0082, 166.4131) (277.1352, 166.5144) (277.2618, 166.6166) (277.388, 166.7196) (277.5137, 166.8235) (277.639, 166.9283) (277.7638, 167.0338) (277.8882, 167.1402) (278.0122, 167.2474) (278.1358, 167.3555) (278.2589, 167.4643) (278.3817, 167.5739) (278.5039, 167.6842) (278.6258, 167.7954) (278.7472, 167.9073) (278.8682, 168.02) (278.9888, 168.1335) (279.1089, 168.2477) (279.2286, 168.3626) (279.3479, 168.4782) (279.4667, 168.5946) (279.5851, 168.7118) (279.7031, 168.8296) (279.8207, 168.9481) (279.9378, 169.0674) (280.0545, 169.1873) (280.1708, 169.3079) (280.2866, 169.4293) (280.402, 169.5512) (280.517, 169.6739) (280.6087, 169.7726) (280.6772, 169.8469) (280.7228, 169.8966) (280.7456, 169.9215) knots 0 0 0 0 0 0 0.01428571 0.02857143 0.04285714 0.05714286 0.07142857 0.08571429 0.1 0.11428571 0.12857143 0.14285714 0.15714286 0.17142857 0.18571429 0.2 0.21428571 0.22857143 0.24285714 0.25714286 0.27142857 0.28571429 0.3 0.31428571 0.32857143 0.34285714 0.35714286 0.37142857 0.38571429 0.4 0.41428571 0.42857143 0.44285714 0.45714286 0.47142857 0.48571429 0.5 0.51428571 0.52857143 0.54285714 0.55714286 0.57142857 0.58571429 0.6 0.61428571 0.62857143 0.64285714 0.65714286 0.67142857 0.68571429 0.7 0.71428571 0.72857143 0.74285714 0.75714286 0.77142857 0.78571429 0.8 0.81428571 0.82857143 0.84285714 0.85714286 0.87142857 0.88571429 0.9 0.91428571 0.92857143 0.94285714 0.95714286 0.97142857 0.98571429 1 1 1 1 1 1
  line L3691 (271.6862, 163.3622) -> (271.7163, 163.369) construction
  line L3692 (271.7163, 163.369) -> (271.7764, 163.3833) construction
  line L3693 (271.7764, 163.3833) -> (271.8658, 163.4071) construction
  line L3694 (271.8658, 163.4071) -> (271.9837, 163.4435) construction
  line L3695 (271.9837, 163.4435) -> (272.1293, 163.4951) construction
  line L3696 (272.1293, 163.4951) -> (272.2736, 163.5511) construction
  line L3697 (272.2736, 163.5511) -> (272.4172, 163.6099) construction
  line L3698 (272.4172, 163.6099) -> (272.5603, 163.6701) construction
  line L3699 (272.5603, 163.6701) -> (272.7031, 163.7313) construction
  line L3700 (272.7031, 163.7313) -> (272.8456, 163.7935) construction
  line L3701 (272.8456, 163.7935) -> (272.9877, 163.8571) construction
  line L3702 (272.9877, 163.8571) -> (273.1291, 163.9226) construction
  line L3703 (273.1291, 163.9226) -> (273.2699, 163.9902) construction
  line L3704 (273.2699, 163.9902) -> (273.4099, 164.06) construction
  line L3705 (273.4099, 164.06) -> (273.5493, 164.1316) construction
  line L3706 (273.5493, 164.1316) -> (273.6881, 164.205) construction
  line L3707 (273.6881, 164.205) -> (273.8264, 164.2797) construction
  line L3708 (273.8264, 164.2797) -> (273.9642, 164.3557) construction
  line L3709 (273.9642, 164.3557) -> (274.1017, 164.4327) construction
  line L3710 (274.1017, 164.4327) -> (274.2387, 164.5109) construction
  line L3711 (274.2387, 164.5109) -> (274.3752, 164.5904) construction
  line L3712 (274.3752, 164.5904) -> (274.5112, 164.6711) construction
  line L3713 (274.5112, 164.6711) -> (274.6468, 164.753) construction
  line L3714 (274.6468, 164.753) -> (274.7818, 164.8363) construction
  line L3715 (274.7818, 164.8363) -> (274.9163, 164.9208) construction
  line L3716 (274.9163, 164.9208) -> (275.0504, 165.0064) construction
  line L3717 (275.0504, 165.0064) -> (275.184, 165.0932) construction
  line L3718 (275.184, 165.0932) -> (275.3172, 165.181) construction
  line L3719 (275.3172, 165.181) -> (275.45, 165.2698) construction
  line L3720 (275.45, 165.2698) -> (275.5823, 165.3597) construction
  line L3721 (275.5823, 165.3597) -> (275.7141, 165.4506) construction
  line L3722 (275.7141, 165.4506) -> (275.8455, 165.5425) construction
  line L3723 (275.8455, 165.5425) -> (275.9765, 165.6354) construction
  line L3724 (275.9765, 165.6354) -> (276.107, 165.7293) construction
  line L3725 (276.107, 165.7293) -> (276.237, 165.8242) construction
  line L3726 (276.237, 165.8242) -> (276.3666, 165.92) construction
  line L3727 (276.3666, 165.92) -> (276.4958, 166.0168) construction
  line L3728 (276.4958, 166.0168) -> (276.6246, 166.1146) construction
  line L3729 (276.6246, 166.1146) -> (276.7529, 166.2132) construction
  line L3730 (276.7529, 166.2132) -> (276.8808, 166.3127) construction
  line L3731 (276.8808, 166.3127) -> (277.0082, 166.4131) construction
  line L3732 (277.0082, 166.4131) -> (277.1352, 166.5144) construction
  line L3733 (277.1352, 166.5144) -> (277.2618, 166.6166) construction
  line L3734 (277.2618, 166.6166) -> (277.388, 166.7196) construction
  line L3735 (277.388, 166.7196) -> (277.5137, 166.8235) construction
  line L3736 (277.5137, 166.8235) -> (277.639, 166.9283) construction
  line L3737 (277.639, 166.9283) -> (277.7638, 167.0338) construction
  line L3738 (277.7638, 167.0338) -> (277.8882, 167.1402) construction
  line L3739 (277.8882, 167.1402) -> (278.0122, 167.2474) construction
  line L3740 (278.0122, 167.2474) -> (278.1358, 167.3555) construction
  line L3741 (278.1358, 167.3555) -> (278.2589, 167.4643) construction
  line L3742 (278.2589, 167.4643) -> (278.3817, 167.5739) construction
  line L3743 (278.3817, 167.5739) -> (278.5039, 167.6842) construction
  line L3744 (278.5039, 167.6842) -> (278.6258, 167.7954) construction
  line L3745 (278.6258, 167.7954) -> (278.7472, 167.9073) construction
  line L3746 (278.7472, 167.9073) -> (278.8682, 168.02) construction
  line L3747 (278.8682, 168.02) -> (278.9888, 168.1335) construction
  line L3748 (278.9888, 168.1335) -> (279.1089, 168.2477) construction
  line L3749 (279.1089, 168.2477) -> (279.2286, 168.3626) construction
  line L3750 (279.2286, 168.3626) -> (279.3479, 168.4782) construction
  line L3751 (279.3479, 168.4782) -> (279.4667, 168.5946) construction
  line L3752 (279.4667, 168.5946) -> (279.5851, 168.7118) construction
  line L3753 (279.5851, 168.7118) -> (279.7031, 168.8296) construction
  line L3754 (279.7031, 168.8296) -> (279.8207, 168.9481) construction
  line L3755 (279.8207, 168.9481) -> (279.9378, 169.0674) construction
  line L3756 (279.9378, 169.0674) -> (280.0545, 169.1873) construction
  line L3757 (280.0545, 169.1873) -> (280.1708, 169.3079) construction
  line L3758 (280.1708, 169.3079) -> (280.2866, 169.4293) construction
  line L3759 (280.2866, 169.4293) -> (280.402, 169.5512) construction
  line L3760 (280.402, 169.5512) -> (280.517, 169.6739) construction
  line L3761 (280.517, 169.6739) -> (280.6087, 169.7726) construction
  line L3762 (280.6087, 169.7726) -> (280.6772, 169.8469) construction
  line L3763 (280.6772, 169.8469) -> (280.7228, 169.8966) construction
  line L3764 (280.7228, 169.8966) -> (280.7456, 169.9215) construction
  arc A110 (269.1057, 157.2806) -> (271.2762, 155.5428) centre (271.0895, 157.5341) ccw
  spline S50 degree 5 poles (252.4583, 104.1847) (252.4787, 104.1615) (252.5188, 104.1146) (252.5771, 104.0427) (252.6512, 103.944) (252.7386, 103.8167) (252.8224, 103.6865) (252.904, 103.5546) (252.9844, 103.4218) (253.064, 103.2883) (253.1427, 103.1542) (253.2203, 103.0193) (253.2962, 102.8832) (253.3703, 102.7457) (253.4426, 102.607) (253.5133, 102.4671) (253.5824, 102.3262) (253.6504, 102.1844) (253.7173, 102.0419) (253.7832, 101.8988) (253.848, 101.755) (253.9118, 101.6105) (253.9744, 101.4653) (254.0359, 101.3193) (254.0962, 101.1726) (254.1554, 101.0251) (254.2135, 100.877) (254.2706, 100.7283) (254.3267, 100.579) (254.3819, 100.4291) (254.4361, 100.2786) (254.4894, 100.1276) (254.5417, 99.976) (254.593, 99.8239) (254.6434, 99.6712) (254.6928, 99.518) (254.7414, 99.3642) (254.789, 99.21) (254.8357, 99.0553) (254.8815, 98.9001) (254.9265, 98.7444) (254.9706, 98.5882) (255.0138, 98.4316) (255.0561, 98.2745) (255.0976, 98.117) (255.1383, 97.9591) (255.1781, 97.8007) (255.217, 97.6419) (255.2551, 97.4827) (255.2924, 97.3231) (255.3289, 97.1631) (255.3646, 97.0027) (255.3994, 96.8419) (255.4335, 96.6807) (255.4667, 96.5191) (255.4992, 96.3572) (255.5308, 96.1949) (255.5617, 96.0323) (255.5917, 95.8693) (255.621, 95.706) (255.6495, 95.5423) (255.6773, 95.3783) (255.7043, 95.2139) (255.7304, 95.0492) (255.7559, 94.8842) (255.7806, 94.7189) (255.8045, 94.5533) (255.8276, 94.3874) (255.85, 94.2211) (255.8717, 94.0546) (255.8926, 93.8878) (255.9087, 93.7541) (255.9205, 93.6537) (255.9282, 93.5867) (255.932, 93.5531) knots 0 0 0 0 0 0 0.01428571 0.02857143 0.04285714 0.05714286 0.07142857 0.08571429 0.1 0.11428571 0.12857143 0.14285714 0.15714286 0.17142857 0.18571429 0.2 0.21428571 0.22857143 0.24285714 0.25714286 0.27142857 0.28571429 0.3 0.31428571 0.32857143 0.34285714 0.35714286 0.37142857 0.38571429 0.4 0.41428571 0.42857143 0.44285714 0.45714286 0.47142857 0.48571429 0.5 0.51428571 0.52857143 0.54285714 0.55714286 0.57142857 0.58571429 0.6 0.61428571 0.62857143 0.64285714 0.65714286 0.67142857 0.68571429 0.7 0.71428571 0.72857143 0.74285714 0.75714286 0.77142857 0.78571429 0.8 0.81428571 0.82857143 0.84285714 0.85714286 0.87142857 0.88571429 0.9 0.91428571 0.92857143 0.94285714 0.95714286 0.97142857 0.98571429 1 1 1 1 1 1
  line L3765 (252.4583, 104.1847) -> (252.4787, 104.1615) construction
  line L3766 (252.4787, 104.1615) -> (252.5188, 104.1146) construction
  line L3767 (252.5188, 104.1146) -> (252.5771, 104.0427) construction
  line L3768 (252.5771, 104.0427) -> (252.6512, 103.944) construction
  line L3769 (252.6512, 103.944) -> (252.7386, 103.8167) construction
  line L3770 (252.7386, 103.8167) -> (252.8224, 103.6865) construction
  line L3771 (252.8224, 103.6865) -> (252.904, 103.5546) construction
  line L3772 (252.904, 103.5546) -> (252.9844, 103.4218) construction
  line L3773 (252.9844, 103.4218) -> (253.064, 103.2883) construction
  line L3774 (253.064, 103.2883) -> (253.1427, 103.1542) construction
  line L3775 (253.1427, 103.1542) -> (253.2203, 103.0193) construction
  line L3776 (253.2203, 103.0193) -> (253.2962, 102.8832) construction
  line L3777 (253.2962, 102.8832) -> (253.3703, 102.7457) construction
  line L3778 (253.3703, 102.7457) -> (253.4426, 102.607) construction
  line L3779 (253.4426, 102.607) -> (253.5133, 102.4671) construction
  line L3780 (253.5133, 102.4671) -> (253.5824, 102.3262) construction
  line L3781 (253.5824, 102.3262) -> (253.6504, 102.1844) construction
  line L3782 (253.6504, 102.1844) -> (253.7173, 102.0419) construction
  line L3783 (253.7173, 102.0419) -> (253.7832, 101.8988) construction
  line L3784 (253.7832, 101.8988) -> (253.848, 101.755) construction
  line L3785 (253.848, 101.755) -> (253.9118, 101.6105) construction
  line L3786 (253.9118, 101.6105) -> (253.9744, 101.4653) construction
  line L3787 (253.9744, 101.4653) -> (254.0359, 101.3193) construction
  line L3788 (254.0359, 101.3193) -> (254.0962, 101.1726) construction
  line L3789 (254.0962, 101.1726) -> (254.1554, 101.0251) construction
  line L3790 (254.1554, 101.0251) -> (254.2135, 100.877) construction
  line L3791 (254.2135, 100.877) -> (254.2706, 100.7283) construction
  line L3792 (254.2706, 100.7283) -> (254.3267, 100.579) construction
  line L3793 (254.3267, 100.579) -> (254.3819, 100.4291) construction
  line L3794 (254.3819, 100.4291) -> (254.4361, 100.2786) construction
  line L3795 (254.4361, 100.2786) -> (254.4894, 100.1276) construction